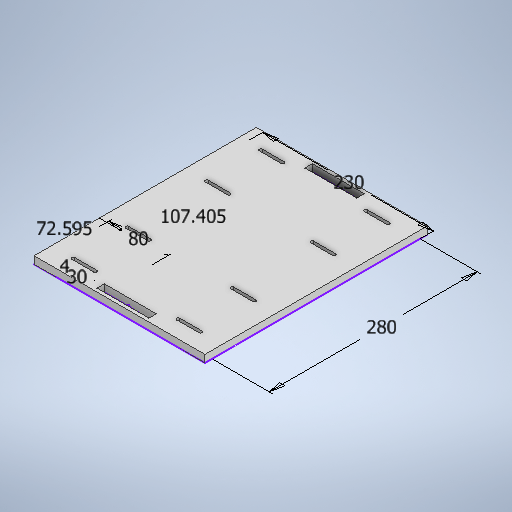
# Autodesk Inventor part: base
Saved by Autodesk Inventor 2025.3 (Build 293356030, 356C)
## iProperties
Created: 2026-06-25
Part Number: base
Material: Generic
Document SubType Name: Modeling
Designer: user
Density: 1 g/cm^3
Appearance: Default
Author: user
Autodesk Inventor part; units mm, degrees
ref_plane "YZ Plane" through (0, 0, 0) normal (1, 0, 0) x (0, 1, 0)
ref_plane "XZ Plane" through (0, 0, 0) normal (0, 1, 0) x (-1, 0, 0)
ref_plane "XY Plane" through (0, 0, 0) normal (0, 0, 1) x (1, 0, 0)
sketch "Sketch1" plane through (0, 0, 0) normal (0, 1, 0) x (-1, 0, 0)
  line L0 (-230, 0) -> (-230, -280)
  line L1 (0, -280) -> (0, 0)
  line L2 (-115, 0) -> (-115, -280) construction
  line L3 (-230, -140) -> (0, -140) construction
  line L4 (0, -230) -> (-230, -230) construction
  line L5 (0, -28.043) -> (0, -96.333) construction
  line L6 (0, -69) -> (0, -31) construction
  line L7 (0, -50) -> (-230, -50) construction
  line L8 (0, -31) -> (-80, -31) construction
  line L9 (-80, -31) -> (-80, -69) construction
  line L10 (-80, -69) -> (0, -69) construction
  line L11 (0, -69) -> (0, -31)
  line L12 (-40, -50) -> (-40, -10.0475) construction
  line L13 (-40, -13.7025) -> (-29.2216, -13.7025)
  line L14 (-40, -13.7025) -> (-59.2216, -13.7025)
  line L15 (-29.2216, -13.7025) -> (-59.2216, -13.7025) construction
  line L16 (-29.2216, -11.7025) -> (-59.2216, -11.7025)
  line L17 (-59.2216, -15.7025) -> (-29.2216, -15.7025)
  arc A0 (-29.2216, -15.7025) -> (-29.2216, -11.7025) centre (-29.2216, -13.7025) ccw
  arc A1 (-59.2216, -11.7025) -> (-59.2216, -15.7025) centre (-59.2216, -13.7025) ccw
  line L18 (-40, -86.2975) -> (-29.2216, -86.2975)
  line L19 (-40, -86.2975) -> (-59.2216, -86.2975)
  line L20 (-29.2216, -86.2975) -> (-59.2216, -86.2975) construction
  line L21 (-29.2216, -88.2975) -> (-59.2216, -88.2975)
  line L22 (-59.2216, -84.2975) -> (-29.2216, -84.2975)
  arc A2 (-29.2216, -88.2975) -> (-29.2216, -84.2975) centre (-29.2216, -86.2975) ccw
  arc A3 (-59.2216, -84.2975) -> (-59.2216, -88.2975) centre (-59.2216, -86.2975) ccw
  line L23 (-230, -31) -> (-150, -31) construction
  line L24 (-150, -31) -> (-150, -69) construction
  line L25 (-150, -69) -> (-230, -69) construction
  line L26 (-190, -13.7025) -> (-200.7784, -13.7025)
  line L27 (-190, -13.7025) -> (-170.7784, -13.7025)
  line L28 (-200.7784, -13.7025) -> (-170.7784, -13.7025) construction
  line L29 (-200.7784, -11.7025) -> (-170.7784, -11.7025)
  line L30 (-170.7784, -15.7025) -> (-200.7784, -15.7025)
  arc A4 (-200.7784, -11.7025) -> (-200.7784, -15.7025) centre (-200.7784, -13.7025) ccw
  arc A5 (-170.7784, -15.7025) -> (-170.7784, -11.7025) centre (-170.7784, -13.7025) ccw
  arc A6 (-170.7784, -88.2975) -> (-170.7784, -84.2975) centre (-170.7784, -86.2975) ccw
  line L31 (-190, -86.2975) -> (-170.7784, -86.2975)
  line L32 (-170.7784, -84.2975) -> (-200.7784, -84.2975)
  line L33 (-190, -86.2975) -> (-200.7784, -86.2975)
  line L34 (-200.7784, -86.2975) -> (-170.7784, -86.2975) construction
  line L35 (-200.7784, -88.2975) -> (-170.7784, -88.2975)
  arc A7 (-200.7784, -84.2975) -> (-200.7784, -88.2975) centre (-200.7784, -86.2975) ccw
  line L36 (-115, -280) -> (-115, 0) construction
  line L37 (0, -230) -> (-230, -230) construction
  line L38 (0, -249) -> (-80, -249) construction
  line L39 (-80, -249) -> (-80, -211) construction
  line L40 (-80, -211) -> (0, -211) construction
  line L41 (-40, -230) -> (-40, -269.9525) construction
  line L42 (-40, -266.2975) -> (-29.2216, -266.2975)
  line L43 (-40, -266.2975) -> (-59.2216, -266.2975)
  line L44 (-29.2216, -266.2975) -> (-59.2216, -266.2975) construction
  line L45 (-29.2216, -268.2975) -> (-59.2216, -268.2975)
  line L46 (-59.2216, -264.2975) -> (-29.2216, -264.2975)
  arc A8 (-29.2216, -268.2975) -> (-29.2216, -264.2975) centre (-29.2216, -266.2975) ccw
  arc A9 (-59.2216, -264.2975) -> (-59.2216, -268.2975) centre (-59.2216, -266.2975) ccw
  arc A10 (-59.2216, -191.7025) -> (-59.2216, -195.7025) centre (-59.2216, -193.7025) ccw
  line L47 (-40, -193.7025) -> (-59.2216, -193.7025)
  line L48 (-59.2216, -195.7025) -> (-29.2216, -195.7025)
  line L49 (-40, -193.7025) -> (-29.2216, -193.7025)
  line L50 (-29.2216, -193.7025) -> (-59.2216, -193.7025) construction
  line L51 (-29.2216, -191.7025) -> (-59.2216, -191.7025)
  arc A11 (-29.2216, -195.7025) -> (-29.2216, -191.7025) centre (-29.2216, -193.7025) ccw
  line L52 (-150, -249) -> (-150, -211) construction
  line L53 (-170.7784, -264.2975) -> (-200.7784, -264.2975)
  line L54 (-190, -266.2975) -> (-200.7784, -266.2975)
  line L55 (-190, -266.2975) -> (-170.7784, -266.2975)
  arc A12 (-200.7784, -264.2975) -> (-200.7784, -268.2975) centre (-200.7784, -266.2975) ccw
  line L56 (-200.7784, -268.2975) -> (-170.7784, -268.2975)
  arc A13 (-170.7784, -268.2975) -> (-170.7784, -264.2975) centre (-170.7784, -266.2975) ccw
  line L57 (-200.7784, -266.2975) -> (-170.7784, -266.2975) construction
  line L58 (-170.7784, -195.7025) -> (-200.7784, -195.7025)
  line L59 (-190, -193.7025) -> (-200.7784, -193.7025)
  arc A14 (-200.7784, -191.7025) -> (-200.7784, -195.7025) centre (-200.7784, -193.7025) ccw
  line L60 (-200.7784, -193.7025) -> (-170.7784, -193.7025) construction
  line L61 (-200.7784, -191.7025) -> (-170.7784, -191.7025)
  line L62 (-190, -193.7025) -> (-170.7784, -193.7025)
  arc A15 (-170.7784, -195.7025) -> (-170.7784, -191.7025) centre (-170.7784, -193.7025) ccw
  line L63 (-150, -211) -> (-230, -211) construction
  line L64 (-230, -249) -> (-150, -249) construction
  line L65 (-192.5048, 9.5806) -> (-30, 9.5806)
  line L66 (-192.5048, -289.5806) -> (-30, -289.5806)
  line L67 (-80, -5) -> (-150, -5)
  line L68 (-150, -5) -> (-150, 5)
  line L69 (-150, 5) -> (-80, 5)
  line L70 (-80, 5) -> (-80, -5)
  line L71 (-80, -275) -> (-150, -275)
  line L72 (-150, -275) -> (-150, -285)
  line L73 (-150, -285) -> (-80, -285)
  line L74 (-80, -285) -> (-80, -275)
  line L75 (0, 0) -> (0, 9.5806)
  line L76 (0, 9.5806) -> (-30, 9.5806)
  line L77 (-192.5048, 9.5806) -> (-230, 9.5806)
  line L78 (-230, 9.5806) -> (-230, 0)
  line L79 (0, -280) -> (0, -289.5806)
  line L80 (0, -289.5806) -> (-30, -289.5806)
  line L81 (-192.5048, -289.5806) -> (-230, -289.5806)
  line L82 (-230, -289.5806) -> (-230, -280)
  point P0 (-40, -31)
  point P1 (-44.2216, -13.7025)
  point P2 (-44.2216, -86.2975)
  point P3 (-190, -50)
  point P4 (-190, -31)
  point P5 (-185.7784, -13.7025)
  point P6 (-185.7784, -86.2975)
  point P7 (-40, -249)
  point P8 (-44.2216, -266.2975)
  point P9 (-44.2216, -193.7025)
  point P10 (-190, -230)
  point P11 (-190, -249)
  point P12 (-185.7784, -193.7025)
  point P13 (-185.7784, -266.2975)
  point P14 (-115, -5)
  point P15 (-44.2216, -86.2975)
  point P16 (-44.2216, -193.7025)
  point P17 (-115, -280)
  point P18 (-115, -280)
  point P19 (-115, -275)
  dimension "d0" = 230
  dimension "d15" = 80
  dimension "d25" = 4
  dimension "d33" = 72.595
  dimension "d34" = 30
  dimension "d35" = 107.405
  dimension "d36" = 280
  constraints: 182 end point, 86 symmetric about line, 32 point on circle, 16 centre point, 12 point on line, 7 midpoint, 6 parallel, 6 perpendicular, 4 horizontal, 4 tangent, 3 collinear, 2 vertical, 14 other
  measures "d0" distance of L1.start L0.end
  measures "d15" distance of L10.end L9.end
  measures "d25" distance of L17.end L16.start
  measures "d33" distance between parallel lines of L17 L21
  measures "d34" distance of L14.end L13.end
  measures "d35" distance of point (-44.222, -193.702) point (-44.222, -86.298)
  measures "d36" distance of L0.start L0.end
extrude "Extrusion1" add sketch "Sketch1" along normal blind 10 contours L78 L77 L65 L76 L75 L1 L79 L80 L66 L81 L82 L0 | A0 L17 A1 L16 | L21 A3 L22 A2 | L29 A5 L30 A4 | L35 A7 L32 A6 | L45 A9 L46 A8 | L51 A11 L48 A10 | A13 L56 A12 L53 | L58 A14 L61 A15 | L67 L68 L69 L70 | L74 L73 L72 L71
extrude "Extrusion2" cut sketch "Sketch1" along normal through all contours A0 L17 A1 L16 | L21 A3 L22 A2 | L29 A5 L30 A4 | L35 A7 L32 A6 | L45 A9 L46 A8 | L51 A11 L48 A10 | A13 L56 A12 L53 | L58 A14 L61 A15
extrude "Extrusion4" add sketch "Sketch1" along normal blind 10 contours L78 L77 L65 L76 L75 L1 L79 L80 L66 L81 L82 L0 | A0 L17 A1 L16 | L21 A3 L22 A2 | L29 A5 L30 A4 | L35 A7 L32 A6 | L45 A9 L46 A8 | L51 A11 L48 A10 | A13 L56 A12 L53 | L58 A14 L61 A15 | L67 L68 L69 L70 | L74 L73 L72 L71
extrude "Extrusion5" cut sketch "Sketch1" along normal blind 10 contours L67 L68 L69 L70 | L74 L73 L72 L71
extrude "Extrusion6" cut sketch "Sketch1" along normal blind 10 contours L29 A5 L30 A4
extrude "Extrusion7" cut sketch "Sketch1" along normal blind 10 contours A0 L17 A1 L16 | L21 A3 L22 A2 | L35 A7 L32 A6 | L45 A9 L46 A8 | L51 A11 L48 A10 | A13 L56 A12 L53 | L58 A14 L61 A15
body "Solid1"
